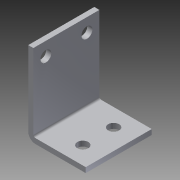
# Autodesk Inventor part: M - Hook Mount Bracket
Saved by Autodesk Inventor 2013 (Build 170138000, 138)
## iProperties
Created: 2013-02-20
Part Number: M - Hook Mount Bracket
Material: Aluminum 6061
Document SubType Name: Sheet Metal
Designer: Moses
Mass: 27.5746 g
Surface Area: 74.5895 cm^2
Volume: 10.1751 cm^3
Density: 2.71 g/cm^3
Sheet Metal Rule: Default
Author: Moses
Autodesk Inventor part; units mm, degrees
ref_plane "YZ Plane" through (0, 0, 0) normal (1, 0, 0) x (0, 1, 0)
ref_plane "XZ Plane" through (0, 0, 0) normal (0, 1, 0) x (-1, 0, 0)
ref_plane "XY Plane" through (0, 0, 0) normal (0, 0, 1) x (1, 0, 0)
sketch "Sketch1" plane through (0, 0, 0) normal (0, 1, 0) x (-1, 0, 0)
  line L0 (0, 0) -> (35.56, 0)
  line L1 (35.56, 0) -> (35.56, 40.8521)
  line L2 (35.56, 40.8521) -> (0, 40.8521)
  line L3 (0, 40.8521) -> (0, 0)
  line L4 (12.7, 29.951) -> (12.7, 10.901) construction
  circle A0 centre (12.7, 29.951) radius 3.3782
  circle A1 centre (12.7, 10.901) radius 3.3782
  line L5 (0, 20.426) -> (35.56, 20.426) construction
  point P0 (12.7, 20.426)
  dimension "d0" = 35.56
  dimension "d2" = 40.8521
  dimension "d3" = 6.7564
  dimension "d4" = 19.05
  dimension "d16" = 12.7
  measures "d0" distance of L1.end L2.end
  measures "d2" distance of L0.end L1.end
  measures "d3" diameter of A0
  measures "d4" distance of L4.start L4.end
  measures "d16" distance between parallel lines of L4 L3
extrude "Plate1" add sketch "Sketch1" along normal blind 3.175
sketch "Sketch2" plane through (-32.385, 0, 40.8521) normal (-1, 0, 0) x (0, -1, 0)
  line L0 (0, -40.8521) -> (0, 0)
  line L1 (0, 0) -> (-50.8, 0)
  line L2 (-50.8, 0) -> (-50.8, -40.8521)
  line L3 (-50.8, -40.8521) -> (0, -40.8521)
  constraints: 6 end point, 1 horizontal, 1 perpendicular, 1 vertical
edge flange "Flange1" height 50.8 angle 90 thickness 3.175 bend radius 1.27 thickness toward (-1, 0, 0) relief straight relief width 3.175 relief depth 1.5875 edges at (-35.56, 3.175, 20.426) wall of the first edge with corners at (-32.385, 0, 0) (-32.385, 0, 40.8521) (-32.385, 50.8, 40.8521) (-32.385, 50.8, 0)
bend "Bend1"
corner "Corner1"
sketch "Sketch3" plane through (-35.56, 50.8, 0) normal (-1, 0, 0) x (0, 0, 1)
  line L0 (0, -46.355) -> (40.8521, -46.355) projected
  line L1 (0, 0) -> (40.8521, 0) projected
  line L2 (0, -46.355) -> (0, 0) projected
  circle A0 centre (7.726, -8.255) radius 3.3782
  circle A1 centre (33.126, -8.255) radius 3.3782
  line L3 (7.726, -8.255) -> (33.126, -8.255) construction
  line L4 (20.426, 0) -> (20.426, -46.355) construction
  point P0 (0, -50.8)
  point P1 (20.426, -8.255)
  dimension "d18" = 6.7564
  dimension "d19" = 38.1
  dimension "d20" = 25.4
  constraints: 4 end point, 3 midpoint, 2 centre point, 1 equal radius, 1 perpendicular, 1 point on line
  measures "d18" diameter of A1
  measures "d19" distance between parallel lines of L0 L3
  measures "d20" distance of L3.start L3.end
extrude "Cut1" cut sketch "Sketch3" against normal blind 3.175
equation "\"d21\" = Thickness"
equation "\"d6\" = BendReliefWidth"
equation "\"d7\" = BendReliefDepth"
equation "\"d8\" = MinimumRemnant"
equation "\"d9\" = BendRadius"
equation "\"d13\" = CornerReliefSize"
equation "\"d14\" = GapSize"
equation "\"d15\" = JacobiRadiusSize"
equation "\"BendRadius\" = Thickness"
equation "\"BendReliefWidth\" = Thickness"
equation "\"BendReliefDepth\" = 0.5 * Thickness"
equation "\"CornerReliefSize\" = 4 * Thickness"
equation "\"MinimumRemnant\" = 2 * Thickness"
equation "\"TransitionRadius\" = BendRadius"
equation "\"JacobiRadiusSize\" = BendRadius"
equation "\"GapSize\" = Thickness"
equation "\"d5\" = BendRadius"
equation "\"Thickness\" = 3.175"
body "Solid1"
